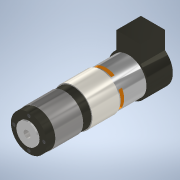
# Autodesk Inventor part: motorbody
Saved by Autodesk Inventor 2020 (Build 240168000, 168)
## iProperties
Created: 2020-07-27
Part Number: motorbody
Material: Steel, Mild
Document SubType Name: Modeling
Designer: Ashiqrahman
Density: 7.85 g/cm^3
Appearance: Semi-Polished
Mass: 1741.14 g
Surface Area: 295.737 cm^2
Volume: 221.801 cm^3
Author: Ashiqrahman
Autodesk Inventor part; units mm, degrees
sketch "Sketch1" plane through (0, 0, 0) normal (0, 0, 1) x (1, 0, 0)
  circle A0 centre (0, 0) radius 20.85
  dimension "d0" = 41.7
  constraints: 1 centre point, 1 coincident
  measures "d0" diameter of A0
extrude "Extrusion1" add sketch "Sketch1" against normal blind 116
ref_plane "Work Plane3" through (0, 0, -44) normal (0, 0, -1) x (-1, 0, 0)
ref_plane "Work Plane2" through (0, 0, -52) normal (0, 0, -1) x (-1, 0, 0)
sketch "Sketch2" plane through (0, 0, -84) normal (0, 0, -1) x (-1, 0, 0)
  circle A0 centre (0, 0) radius 20.85 projected
  circle A1 centre (0, 0) radius 21
  dimension "d6" = 42
  constraints: 1 centre point, 1 coincident
  measures "d6" diameter of A1
extrude "Extrusion2" add sketch "Sketch2" along normal up to surface (32 mm away)
sketch "Sketch3" plane through (0, 0, -84) normal (0, 0, -1) x (-1, 0, 0)
  circle A0 centre (0, 0) radius 22
  circle A1 centre (0, 0) radius 20.85 projected
  dimension "d9" = 44
  constraints: 1 centre point, 1 coincident
  measures "d9" diameter of A0
extrude "Extrusion3" add sketch "Sketch3" against normal up to surface (32 mm away)
sketch "Sketch4" plane through (0, 0, 0) normal (0, 0, 1) x (1, 0, 0)
  circle A0 centre (0, 0) radius 17.5
  circle A1 centre (0, 17.5) radius 2
  circle A2 centre (-17.5, 0) radius 2
  circle A3 centre (0, -17.5) radius 2
  circle A4 centre (17.5, 0) radius 2
  dimension "d12" = 35
  dimension "d13" = 4
  dimension "d16" = 360
  constraints: 4 centre point, 1 coincident, 1 vertical alignment, 11 other
  measures "d13" diameter of A1
extrude "Extrusion4" cut sketch "Sketch4" against normal blind 6 contours A0 A4 | A0 A4 | A1 A0 | A0 A1 | A3 A0 | A0 A3 | A2 A0 | A0 A2
sketch "Sketch5" plane through (0, 0, 0) normal (0, 0, 1) x (1, 0, 0)
  circle A0 centre (0, 0) radius 12.5
  dimension "d20" = 25
  constraints: 1 centre point, 1 coincident
  measures "d20" diameter of A0
extrude "Extrusion5" add sketch "Sketch5" along normal blind 2
sketch "Sketch6" plane through (0, 0, 2) normal (0, 0, 1) x (1, 0, 0)
  circle A0 centre (0, 0) radius 4
  dimension "d23" = 8
  constraints: 1 centre point, 1 coincident
  measures "d23" diameter of A0
extrude "Extrusion6" cut sketch "Sketch6" against normal up to surface (46 mm away)
sketch "Sketch7" plane through (0, 0, -116) normal (0, 0, -1) x (-1, 0, 0)
  circle A0 centre (0, 0) radius 23.25
  circle A1 centre (0, 0) radius 21 projected
  dimension "d26" = 46.5
  dimension "d27" = 42
  constraints: 1 centre point, 1 coincident
  measures "d26" diameter of A0
  measures "d27" diameter of A1
extrude "Extrusion7" add sketch "Sketch7" along normal blind 28.5 contours A0 | A1
ref_plane "Work Plane4" through (0, 17.5, 0) normal (0, 1, 0) x (-1, 0, 0)
sketch "Sketch8" plane through (0, 17.5, 0) normal (0, 1, 0) x (-1, 0, 0)
  line L0 (-23.25, -144.5) -> (23.25, -144.5) projected
  line L1 (-23.25, -116) -> (23.25, -116) projected
  line L2 (-23.25, -116) -> (23.25, -116) projected
  line L3 (-23.25, -144.5) -> (23.25, -144.5) projected
  line L4 (23.25, -116) -> (-23.25, -144.5)
  line L5 (-14, -116) -> (14, -116)
  line L6 (14, -116) -> (14, -144.5)
  line L7 (14, -144.5) -> (-14, -144.5)
  line L8 (-14, -144.5) -> (-14, -116)
  line L9 (-14, -116) -> (14, -144.5) construction
  line L10 (14, -116) -> (-14, -144.5) construction
  point P0 (0, 0)
  point P1 (0, -130.25)
  dimension "d31" = 28
  constraints: 14 end point, 3 midpoint, 2 parallel, 1 horizontal, 1 perpendicular, 1 point on line
  measures "d31" distance of L6.end L7.end
extrude "Extrusion8" add sketch "Sketch8" along normal blind 21.5 contours L8 L4 L6 L0 | L8 L1 L6 L4
ref_plane "Work Plane5" through (0, 0, -42) normal (0, 0, 1) x (1, 0, 0)
ref_plane "Work Plane6" through (0, 0, -10) normal (0, 0, 1) x (1, 0, 0)
sketch "Sketch9" plane through (0, 0, -10) normal (0, 0, 1) x (1, 0, 0)
  circle A0 centre (0, 0) radius 12.5 projected
  circle A1 centre (-17.5, 0) radius 2 projected
  circle A2 centre (0, 17.5) radius 2 projected
  circle A3 centre (0, -17.5) radius 2 projected
  circle A4 centre (17.5, 0) radius 2 projected
  circle A5 centre (0, 0) radius 20.85 projected
  circle A6 centre (0, 0) radius 4 projected
  circle A7 centre (0, 0) radius 21.35
  dimension "d36" = 42.7
  constraints: 1 centre point, 1 coincident
  measures "d36" diameter of A7
extrude "Extrusion9" add sketch "Sketch9" against normal up to surface (32 mm away) contours A7
ref_plane "Work Plane7" through (0, 21, 0) normal (0, 1, 0) x (-1, 0, 0)
sketch "Sketch10" plane through (0, 21, 0) normal (0, 1, 0) x (-1, 0, 0)
  line L0 (-21, -84) -> (21, -84) projected
  line L1 (-21, -116) -> (21, -116) projected
  line L2 (-21, -84) -> (21, -84) projected
  line L3 (0, -84) -> (0, -88)
  line L4 (-10, -90) -> (10, -90)
  line L5 (10, -90) -> (10, -86)
  line L6 (10, -86) -> (-10, -86)
  line L7 (-10, -86) -> (-10, -90)
  line L8 (-10, -90) -> (10, -86) construction
  line L9 (10, -90) -> (-10, -86) construction
  point P0 (0, 0)
  dimension "d40" = 4
  dimension "d41" = 20
  dimension "d42" = 4
  constraints: 14 end point, 3 midpoint, 2 parallel, 1 horizontal, 1 perpendicular, 1 vertical
  measures "d40" distance of L3.start L3.end
  measures "d41" distance of L6.end L5.end
  measures "d42" distance of L5.end L4.end
extrude "Extrusion10" cut sketch "Sketch10" against normal through all
pattern_circular "Circular Pattern1" count 2 over 90 about axis through (0, 0, -84) along (0, 0, -1) of "Extrusion10"
thread "Thread1" size "M4x0.7" class "6H" standard "ANSI Metric M Profile" length 146
thread "Thread2" size "M4x0.7" class "6H" standard "ANSI Metric M Profile" length 146
thread "Thread3" size "M4x0.7" class "6H" standard "ANSI Metric M Profile" length 146
thread "Thread4" size "M4x0.7" class "6H" standard "ANSI Metric M Profile" length 146
ref_plane "Work Plane1" through (0, 0, -84) normal (0, 0, -1) x (-1, 0, 0)
body "Solid1"
